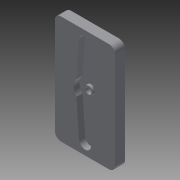
# Autodesk Inventor part: arm-slot
Saved by Autodesk Inventor 2015 (Build 190159000, 159)
## iProperties
Created: 2014-07-18
Part Number: arm-slot
Material: Generic
Document SubType Name: Modeling
Designer: pc
Density: 1 g/cm^3
Appearance: Default
Author: pc
Autodesk Inventor part; units mm, degrees
ref_plane "YZ Plane" through (0, 0, 0) normal (1, 0, 0) x (0, 1, 0)
ref_plane "XZ Plane" through (0, 0, 0) normal (0, 1, 0) x (-1, 0, 0)
ref_plane "XY Plane" through (0, 0, 0) normal (0, 0, 1) x (1, 0, 0)
sketch "Sketch1" plane through (0, 0, 0) normal (0, 1, 0) x (-1, 0, 0)
  line L0 (9.98, 17.98) -> (-9.98, 17.98)
  line L1 (-9.98, 17.98) -> (-9.98, -17.98)
  line L2 (-9.98, -17.98) -> (9.98, -17.98)
  line L3 (9.98, -17.98) -> (9.98, 17.98)
  line L4 (9.98, 17.98) -> (-9.98, -17.98) construction
  line L5 (-9.98, 17.98) -> (9.98, -17.98) construction
  point P0 (0, 0)
  dimension "d0" = 35.96
  dimension "d1" = 19.96
  constraints: 12 end point, 2 midpoint, 2 parallel, 1 horizontal, 1 perpendicular
  measures "d0" distance of L0.end L1.end
  measures "d1" distance of L0.start L0.end
extrude "arm-horn" add sketch "Sketch1" along normal blind 3.3
fillet "Fillet1" radius 2 1 edges at (-9.98, 1.65, 17.98)
fillet "Fillet2" radius 2 1 edges at (9.98, 1.65, 17.98)
fillet "Fillet3" radius 2 1 edges at (9.98, 1.65, -17.98)
fillet "Fillet4" radius 2 1 edges at (-9.98, 1.65, -17.98)
sketch "Sketch3" plane through (0, 0, 0) normal (0, -1, 0) x (1, 0, 0)
  arc A0 (-2.612, 2.76) -> (-2.8345, 2.5309) centre (0, 0) ccw construction
  arc A1 (-1.9951, -14.4406) -> (1.9951, -14.4406) centre (0, -14.3) ccw
  arc A2 (0, 12.3) -> (1.9951, 14.4406) centre (0, 14.3) ccw construction
  line L0 (1.9951, 14.4406) -> (2.8345, 2.5309)
  line L1 (-1.9951, 14.4406) -> (-2.8345, 2.5309)
  line L2 (-2.8345, -2.5309) -> (-1.9951, -14.4406)
  line L3 (2.8345, -2.5309) -> (1.9951, -14.4406)
  circle A3 centre (0, -1.5) radius 2.9 construction
  arc A4 (-2.612, 2.76) -> (-2.8928, 1.7039) centre (0, 1.5) ccw construction
  line L4 (-7.98, 17.98) -> (7.98, 17.98) construction
  line L5 (0, 17.98) -> (0, -18.0608) construction
  line L6 (7.98, -17.98) -> (-7.98, -17.98) construction
  arc A5 (0, 4.4) -> (-2.612, 2.76) centre (0, 1.5) ccw construction
  arc A6 (2.612, 2.76) -> (0, 4.4) centre (0, 1.5) ccw construction
  arc A7 (0, 3.8) -> (-2.612, 2.76) centre (0, 0) ccw construction
  arc A8 (2.612, 2.76) -> (0, 3.8) centre (0, 0) ccw construction
  arc A9 (-2.8928, 1.7039) -> (-2.4819, 0) centre (0, 1.5) ccw construction
  arc A10 (-2.4819, 0) -> (2.4819, 0) centre (0, 1.5) ccw construction
  arc A11 (2.4819, 0) -> (2.8928, 1.7039) centre (0, 1.5) ccw construction
  arc A12 (2.8928, 1.7039) -> (2.612, 2.76) centre (0, 1.5) ccw construction
  line L7 (-2.8345, 2.5309) -> (-2.8928, 1.7039) construction
  arc A13 (-2.8345, 2.5309) -> (-2.8345, -2.5309) centre (0, 0) ccw
  arc A14 (0, -3.8) -> (2.612, -2.76) centre (0, 0) ccw construction
  arc A15 (-2.612, -2.76) -> (0, -3.8) centre (0, 0) ccw construction
  arc A16 (2.612, -2.76) -> (2.8345, -2.5309) centre (0, 0) ccw construction
  arc A17 (-2.8345, -2.5309) -> (-2.612, -2.76) centre (0, 0) ccw construction
  arc A18 (2.8345, -2.5309) -> (2.612, 2.76) centre (0, 0) ccw
  arc A19 (-1.9951, 14.4406) -> (0, 12.3) centre (0, 14.3) ccw construction
  arc A20 (1.9951, 14.4406) -> (-1.9951, 14.4406) centre (0, 14.3) ccw
  arc A21 (0, -12.3) -> (-1.9951, -14.4406) centre (0, -14.3) ccw construction
  arc A22 (1.9951, -14.4406) -> (0, -12.3) centre (0, -14.3) ccw construction
  line L8 (2.8345, 2.5309) -> (2.8928, 1.7039) construction
  point P0 (0, -17.98)
  dimension "d12" = 4
  dimension "d13" = 5.8
  dimension "d14" = 7.6
  dimension "d16" = 1.5
  dimension "d17" = 1.5
  dimension "d18" = 14.3
  dimension "d19" = 14.3
  constraints: 62 point on circle, 34 tangent, 23 centre point, 12 end point, 2 coincident, 2 equal radius, 2 horizontal, 2 midpoint, 13 other
  measures "d12" diameter of A1
  measures "d13" diameter of A3
  measures "d14" diameter of A0
  measures "d16" distance of A0.centre A4.centre
  measures "d17" distance of point (0, 0) A3.centre
  measures "d18" distance of point (0, 0) A1.centre
  measures "d19" distance of A2.centre point (0, 0)
extrude "Extrusion3" cut sketch "Sketch3" against normal blind 2
sketch "Sketch6" plane through (0, 3.3, 0) normal (0, 1, 0) x (1, 0, 0)
  circle A0 centre (0, 0) radius 1
  circle A1 centre (0, 0) radius 1.5
  dimension "d29" = 2
  dimension "d30" = 3
  constraints: 2 centre point, 2 coincident
  measures "d29" diameter of A0
  measures "d30" diameter of A1
extrude "Extrusion6" add sketch "Sketch6" against normal blind 2.2
sketch "Sketch7" plane through (0, 3.3, 0) normal (0, 1, 0) x (1, 0, 0)
  circle A0 centre (0, 0) radius 2.5
  dimension "d33" = 5
  constraints: 1 centre point, 1 coincident
  measures "d33" diameter of A0
extrude "Extrusion7" cut sketch "Sketch7" against normal blind 1
sketch "Sketch8" plane through (0, 2.3, 0) normal (0, 1, 0) x (1, 0, 0)
  circle A0 centre (0, 0) radius 1
  dimension "d36" = 2
  constraints: 1 centre point, 1 coincident
  measures "d36" diameter of A0
extrude "Extrusion8" cut sketch "Sketch8" against normal up to next
equation "\"d8\" = cornerrad"
equation "\"d9\" = cornerrad"
equation "\"d10\" = cornerrad"
equation "\"d11\" = cornerrad"
equation "\"d19\" = d18"
equation "\"d20\" = armslotd"
equation "\"printer3dtolerance\" = 0.12"
equation "\"wallw\" = 42"
equation "\"wallh\" = 44"
equation "\"cornerrad\" = 2"
equation "\"baseextra\" = 2"
equation "\"wall1_thick\" = 8"
equation "\"wall2_thick\" = 6.4"
equation "\"wall3_thick\" = 4"
equation "\"wall1slot\" = 8.12"
equation "\"wall2slot\" = 6.52"
equation "\"wall3slot\" = 4.12"
equation "\"gap2\" = 28"
equation "\"baseh\" = 79.12"
equation "\"basew\" = 44"
equation "\"base_thick\" = 6"
equation "\"base_slots_depth\" = 4"
equation "\"servobigcircledia\" = 11.62"
equation "\"servosmallcircledia\" = 5.92"
equation "\"servo9gw\" = 22.8"
equation "\"servomounth\" = 4"
equation "\"servomountsquare\" = 4"
equation "\"servopolygonr\" = 6.12"
equation "\"servopolygonl\" = 5.92"
equation "\"distancefrombottom\" = 34"
equation "\"distancefromleft\" = 26"
equation "\"wall3slotd\" = 2"
equation "\"wall3slotw\" = 36"
equation "\"adapterh\" = 16"
equation "\"adapterw\" = 32"
equation "\"armw\" = 36"
equation "\"armslotd\" = 2"
equation "\"armthick\" = 3"
equation "\"fanhs\" = 9.6"
equation "\"fanhb\" = 11"
equation "\"adapterwallthick\" = 6"
equation "\"adapterwallslotd\" = 2"
equation "\"armhornthick\" = 3"
equation "\"hornscrewholed\" = 2"
equation "\"hornthick\" = 1.5"
equation "\"hornscrewheadd\" = 3"
body "Solid1"
